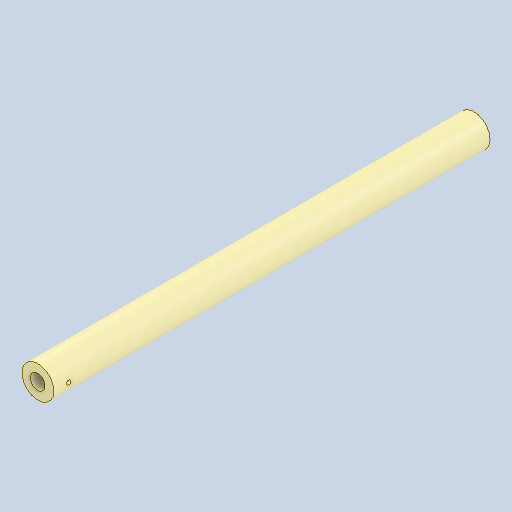
# Autodesk Inventor part: shaft
Saved by Autodesk Inventor 2023 (Build 270158000, 158)
## iProperties
Created: 2022-06-05
Part Number: shaft
Material: Nylon 6/6
Document SubType Name: Modeling
Designer: prana_p9lsmih
Density: 1.13 g/cm^3
Appearance: Nylon 6
Mass: 31.997 g
Surface Area: 144.851 cm^2
Volume: 28.3159 cm^3
Author: prana_p9lsmih
Autodesk Inventor part; units mm, degrees
ref_plane "XZ Plane" through (0, 0, 0) normal (0, 1, 0) x (-1, 0, 0)
ref_plane "XY Plane" through (0, 0, 0) normal (0, 0, 1) x (1, 0, 0)
sketch "Sketch1" plane through (0, 0, 0) normal (0, 0, 1) x (1, 0, 0)
  circle A0 centre (0, 0) radius 7.5
  dimension "d0" = 15
  constraints: 1 centre point, 1 coincident
  measures "d0" diameter of A0
extrude "Extrusion1" add sketch "Sketch1" along normal blind 205.029
sketch "Sketch2" plane through (0, 0, 205.029) normal (0, 0, 1) x (1, 0, 0)
  point P0 (0, 0)
  point P1 (-0.1268, -0.0213)
hole "Hole1" at (-0.1268, -0.0213, 205.029) direction (0, 0, -1) diameter 7 end through all
ref_plane "Work Plane1" through (7.5, 0, 0) normal (1, 0, 0) x (0, 1, 0)
sketch "Sketch3" plane through (7.5, 0, 0) normal (1, 0, 0) x (0, 1, 0)
  circle A0 centre (0, 198.029) radius 1
  line L0 (7.5, 205.029) -> (-7.5, 205.029) projected
  point P0 (0, 0)
  dimension "d10" = 2
  dimension "d11" = 7
  constraints: 1 centre point
  measures "d10" diameter of A0
  measures "d11" distance from line of A0.centre L0
extrude "Extrusion2" cut sketch "Sketch3" against normal through all
body "Solid1"
